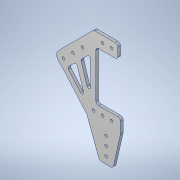
# Autodesk Inventor part: オムニ_後ろ側板
Saved by Autodesk Inventor 2021 (Build 250183000, 183)
## iProperties
Created: 2021-12-02
Part Number: オムニ_後ろ側板
Material: アルミニウム 6061
Document SubType Name: Modeling
Designer: 堀川皓史
Density: 2.7 g/cm^3
Appearance: アルミニウム - フラット
Author: 堀川皓史
Autodesk Inventor part; units mm, degrees
ref_plane "YZ Plane" through (0, 0, 0) normal (1, 0, 0) x (0, 1, 0)
ref_plane "XZ Plane" through (0, 0, 0) normal (0, 1, 0) x (-1, 0, 0)
ref_plane "XY Plane" through (0, 0, 0) normal (0, 0, 1) x (1, 0, 0)
sketch "スケッチ1" plane through (0, 0, 0) normal (0, 0, 1) x (1, 0, 0)
  line L0 (67.5, 17.5) -> (-67.5, 17.5) construction
  line L1 (-67.5, 17.5) -> (-67.5, -17.5) construction
  line L2 (-67.5, -17.5) -> (67.5, -17.5) construction
  line L3 (67.5, -17.5) -> (67.5, 17.5) construction
  line L4 (67.5, 17.5) -> (-67.5, -17.5) construction
  line L5 (-67.5, 17.5) -> (67.5, -17.5) construction
  circle A0 centre (-60, 35) radius 1.6
  circle A1 centre (-70, 35) radius 1.6
  line L6 (-77.5, 27.5) -> (-53, 27.5)
  line L7 (-53, 27.5) -> (-53, 42.5)
  line L8 (-53, 42.5) -> (-80, 42.5) construction
  line L9 (-77.5, 27.5) -> (-77.5, -27.5)
  line L10 (-77.5, -27.5) -> (-50, -27.5)
  circle A2 centre (-60, -35) radius 1.6
  circle A3 centre (-70, -35) radius 1.6
  circle A4 centre (-80, -35) radius 1.6
  line L11 (124.2308, -31.7536) -> (484.5935, -392.1164)
  line L12 (484.5935, -392.1164) -> (488.7129, -553.575)
  line L13 (-80, 21.2868) -> (-468.838, -367.5512) construction
  line L14 (-468.838, -367.5512) -> (-479.4446, -356.9446)
  line L15 (-479.4446, -356.9446) -> (-90.6066, 31.8934) construction
  line L16 (-90.6066, 31.8934) -> (-80, 21.2868) construction
  line L17 (-80, 42.5) -> (-80, 5.3052) construction
  circle A5 centre (-92.3744, 19.519) radius 1.6
  circle A6 centre (-102.981, 8.9124) radius 1.6
  circle A7 centre (-113.5876, -1.6942) radius 1.6
  line L18 (-92.3744, 19.519) -> (-113.5876, -1.6942) construction
  circle A8 centre (-433.75, -321.8566) radius 1.6
  circle A9 centre (-421.9492, -310.0558) radius 1.6
  line L19 (-388.4374, -772.2067) -> (-358.1265, -754.7067) construction
  line L20 (-358.1265, -754.7067) -> (-425.6265, -637.7933) construction
  line L21 (-455.9374, -655.2933) -> (-358.1265, -754.7067) construction
  line L22 (-388.4374, -772.2067) -> (-425.6265, -637.7933) construction
  line L23 (-455.9374, -655.2933) -> (-388.4374, -772.2067) construction
  line L24 (-425.6265, -637.7933) -> (-455.9374, -655.2933) construction
  line L25 (455.9374, -655.2933) -> (425.6265, -637.7933) construction
  line L26 (425.6265, -637.7933) -> (358.1265, -754.7067) construction
  line L27 (388.4374, -772.2067) -> (425.6265, -637.7933) construction
  line L28 (455.9374, -655.2933) -> (358.1265, -754.7067) construction
  line L29 (388.4374, -772.2067) -> (455.9374, -655.2933) construction
  line L30 (358.1265, -754.7067) -> (388.4374, -772.2067) construction
  line L31 (0, 0) -> (0, -263.4473) construction
  line L32 (67.5, 17.5) -> (67.5, -17.5) construction
  circle A10 centre (60, 35) radius 1.6
  circle A11 centre (70, 35) radius 1.6
  line L33 (77.5, 27.5) -> (53, 27.5)
  line L34 (53, 27.5) -> (53, 42.5)
  line L35 (53, 42.5) -> (80, 42.5)
  line L36 (77.5, 27.5) -> (77.5, -27.5)
  line L37 (77.5, -27.5) -> (50, -27.5)
  line L38 (50, -27.5) -> (72.3664, -42.5)
  line L39 (72.3664, -42.5) -> (99.3664, -42.5)
  circle A12 centre (60, -35) radius 1.6
  circle A13 centre (70, -35) radius 1.6
  circle A14 centre (80, -35) radius 1.6
  line L40 (80, 42.5) -> (80, 5.3052) construction
  line L41 (-483.838, -367.5512) -> (-468.838, -367.5512)
  line L42 (-468.838, -367.5512) -> (-468.838, -648.3077)
  line L43 (-468.838, -648.3077) -> (-483.838, -648.3077)
  line L44 (-483.838, -648.3077) -> (-483.838, -367.5512)
  line L45 (-283.2277, -604.4352) -> (-262.2277, -640.8083) construction
  line L46 (345.2492, -497.0108) -> (305.7786, -565.3759) construction
  line L47 (265.1134, -631.6538) -> (-234.8866, -631.6538) construction
  line L48 (-234.8866, -631.6538) -> (-234.8866, -1131.6538) construction
  line L49 (-234.8866, -1131.6538) -> (265.1134, -1131.6538) construction
  line L50 (265.1134, -1131.6538) -> (265.1134, -631.6538) construction
  line L51 (265.1134, -631.6538) -> (-234.8866, -1131.6538) construction
  line L52 (-234.8866, -631.6538) -> (265.1134, -1131.6538) construction
  line L53 (-12.841, -157.5) -> (15.1134, -157.5) construction
  circle A15 centre (1.1362, -409.4569) radius 212.5 construction
  line L54 (501.1362, 53.616) -> (-498.8638, 53.616) construction
  line L55 (-498.8638, 53.616) -> (-498.8638, -946.384) construction
  line L56 (-498.8638, -946.384) -> (501.1362, -946.384) construction
  line L57 (501.1362, -946.384) -> (501.1362, 53.616) construction
  line L58 (501.1362, 53.616) -> (-498.8638, -946.384) construction
  line L59 (-498.8638, 53.616) -> (501.1362, -946.384) construction
  circle A16 centre (1.1362, -409.4569) radius 250 construction
  line L60 (-80, 42.5) -> (-90.6066, 31.8934) construction
  line L61 (-80, 42.5) -> (-118.8909, 3.6091)
  line L62 (-118.8909, -6.9975) -> (-113.5876, -12.3008)
  line L63 (-113.5876, -12.3008) -> (-87.5, -42.5)
  arc A17 (-118.8909, 3.6091) -> (-118.8909, -6.9975) centre (-113.5876, -1.6942) ccw
  line L64 (-80, 42.5) -> (-53, 42.5)
  circle A18 centre (-66, -52.5) radius 1.6
  circle A19 centre (-66, -62.5) radius 1.6
  circle A20 centre (-66, -72.5) radius 1.6
  line L65 (-58.5, -80) -> (-73.5, -80)
  line L66 (-73.5, -80) -> (-87.5, -42.5)
  line L67 (-50, -27.5) -> (-50, -42.5)
  line L68 (-50, -42.5) -> (-58.5, -80)
  point P0 (0, -470)
  point P1 (-102.981, 8.9124)
  point P2 (-77.5, 0)
  point P3 (-407.0319, -705)
  point P4 (-407.0319, -705)
  point P5 (407.0319, -705)
  point P6 (407.0319, -705)
  point P7 (77.5, 0)
  point P8 (15.1134, -881.6538)
  point P9 (1.1362, -446.384)
  point P10 (-124.1942, -1.6942)
  dimension "d27" = 135
  dimension "d28" = 35
  dimension "d29" = 3.2
  dimension "d30" = 3.2
  dimension "d31" = 10
  dimension "d32" = 15
  dimension "d33" = 10
  dimension "d34" = 7.5
  dimension "d35" = 7
  dimension "d36" = 70
  dimension "d37" = 3.2
  dimension "d38" = 3.2
  dimension "d39" = 3.2
  dimension "d40" = 10
  dimension "d41" = 10
  dimension "d45" = 10
  dimension "d46" = 10
  dimension "d53" = 135
  dimension "d54" = 15
  dimension "d55" = 10
  dimension "d57" = 3.2
  dimension "d58" = 3.2
  dimension "d59" = 3.2
  dimension "d60" = 10
  dimension "d61" = 15
  dimension "d62" = 15
  dimension "d63" = 7.5
  dimension "d64" = 45
  dimension "d65" = 3.2
  dimension "d66" = 3.2
  dimension "d69" = 360
  dimension "d76" = 470
  dimension "d77" = 15
  dimension "d80" = 500
  dimension "d81" = 500
  dimension "d82" = 200
  dimension "d83" = 425
  dimension "d84" = 1000
  dimension "d85" = 1000
  dimension "d88" = 42
  dimension "d89" = 500
  dimension "d90" = 7.5
  dimension "d91" = 7.5
  dimension "d112" = 3.2
  dimension "d113" = 3.2
  dimension "d114" = 3.2
  dimension "d115" = 10
  dimension "d116" = 10
  dimension "d117" = 25
  dimension "d118" = 66
  dimension "d120" = 7.5
  dimension "d121" = 7.5
  dimension "d122" = 7.5
  dimension "d123" = 7.5
  dimension "d124" = 7.5
  dimension "d129" = 10
  dimension "d130" = 7.5
  dimension "d131" = 7.5
  constraints: 138 end point, 21 centre point, 14 midpoint, 14 symmetric about line, 11 parallel, 9 perpendicular, 8 horizontal, 5 point on line, 4 vertical, 4 vertical alignment, 3 coincident, 3 horizontal alignment, 2 point on circle, 2 tangent, 1 collinear, 42 other
  measures "d27" distance of L2.end L1.end
  measures "d28" distance of L1.end L0.end
  measures "d29" diameter of A0
  measures "d30" diameter of A1
  measures "d31" distance of A0.centre A1.centre
  measures "d32" distance between parallel lines of L6 L8
  measures "d33" distance between parallel lines of L0 L6
  measures "d34" distance from line of L6 A0.centre
  measures "d35" distance from line of L7 A0.centre
  measures "d36" horizontal distance of A1.centre point (0, 0)
  measures "d37" diameter of A2
  measures "d38" diameter of A3
  measures "d39" diameter of A4
  measures "d40" distance of A3.centre A4.centre
  measures "d41" distance of A2.centre A3.centre
  measures "d45" distance between parallel lines of L10 L2
  measures "d46" distance between parallel lines of L9 L1
  measures "d53" angle of L2 L11
  measures "d54" distance of L13.end L14.end
  measures "d55" distance from line of A1.centre L17
  measures "d57" diameter of A5
  measures "d58" diameter of A6
  measures "d59" diameter of A7
  measures "d60" distance from line of L16 L18.start
  measures "d61" distance of A6.centre L18.start
  measures "d62" distance of L18.end A6.centre
  measures "d63" distance between parallel lines of L13 L18
  measures "d64" angle of L9 L13
  measures "d65" diameter of A8
  measures "d66" diameter of A9
  measures "d76" distance of point (0, -470) point (-407.032, -705)
  measures "d77" distance of L42.end L43.end
  measures "d80" distance of L49.end L48.end
  measures "d81" distance of L48.end L47.end
  measures "d82" distance from line of L53.end L8
  measures "d83" diameter of A15
  measures "d84" distance of L56.end L55.end
  measures "d85" distance of L55.end L54.end
  measures "d88" distance of L45.start L45.end
  measures "d89" diameter of A16
  measures "d90" distance from line of L62 L18.end
  measures "d91" radius of A17
  measures "d112" diameter of A18
  measures "d113" diameter of A19
  measures "d114" diameter of A20
  measures "d115" distance of A19.centre A18.centre
  measures "d116" distance of A20.centre A19.centre
  measures "d117" distance from line of L10 A18.centre
  measures "d118" distance from line of L31 A18.centre
  measures "d120" distance from line of A20.centre L65
  measures "d121" horizontal distance of L63.end A4.centre
  measures "d122" horizontal distance of A4.centre L63.end
  measures "d123" distance from line of L10 A4.centre
  measures "d124" horizontal distance of A20.centre L65.end
  measures "d129" distance from line of A2.centre L67
  measures "d130" horizontal distance of A20.centre L65.start
  measures "d131" vertical distance of A2.centre L67.end
extrude "押し出し1" add sketch "スケッチ1" along normal blind 3 contours L9 L10 L67 L68 L65 L66 L63 L62 A17 L61 L64 L7 L6
fillet "フィレット1" radius 3 10 edges at (-113.5876, -12.3008, 1.5) (-50, -27.5, 1.5) (-77.5, -27.5, 1.5) (-77.5, 27.5, 1.5) (-53, 27.5, 1.5) (-53, 42.5, 1.5) (-80, 42.5, 1.5) (-87.5, -42.5, 1.5) (-73.5, -80, 1.5) (-58.5, -80, 1.5)
sketch "スケッチ2" plane through (0, 0, 3) normal (0, 0, 1) x (1, 0, 0)
  line L0 (-108.1182, -9.4538) -> (-94.6826, -25.0069)
  line L1 (-83.5, -14.6862) -> (-83.5, 12.9584)
  line L2 (-86.9142, 14.3726) -> (-93.4726, 7.8142)
  line L3 (-77.5, -24.5) -> (-77.5, 24.5) projected
  line L4 (-80.8787, 41.6213) -> (-118.8909, 3.6091) projected
  line L5 (-113.516, -12.3836) -> (-87.852, -42.0925) projected
  line L6 (-96.7234, 4.5634) -> (-83.5, -37.9521) construction
  line L7 (-98.1366, -0.994) -> (-91.2594, -23.1055)
  line L8 (-93.9681, 5.806) -> (-87.4098, -15.2802)
  line L9 (-101.4606, -0.1738) -> (-108.019, -6.7322)
  arc A0 (-98.1366, -0.994) -> (-101.4606, -0.1738) centre (-100.0464, -1.588) ccw
  arc A1 (-93.4726, 7.8142) -> (-93.9681, 5.806) centre (-92.0583, 6.4) ccw
  arc A2 (-94.6826, -25.0069) -> (-91.2594, -23.1055) centre (-93.1692, -23.6995) ccw
  arc A3 (-87.4098, -15.2802) -> (-83.5, -14.6862) centre (-85.5, -14.6862) ccw
  arc A4 (-83.5, 12.9584) -> (-86.9142, 14.3726) centre (-85.5, 12.9584) ccw
  arc A5 (-108.019, -6.7322) -> (-108.1182, -9.4538) centre (-106.6047, -8.1464) ccw
  line L10 (-53, -27.5) -> (-74.5, -27.5) projected
  point P0 (0, 0)
  point P1 (-99.1198, 2.167)
  dimension "d95" = 6
  dimension "d97" = 15
  dimension "d98" = 6
  dimension "d99" = 3
  dimension "d100" = 3
  dimension "d101" = 2
  dimension "d102" = 2
  constraints: 14 end point, 12 point on circle, 12 tangent, 7 point on line, 6 centre point, 5 parallel, 4 equal radius, 1 collinear, 1 vertical
  measures "d95" distance between parallel lines of L3 L1
  measures "d97" distance between parallel lines of L4 L2
  measures "d98" distance between parallel lines of L5 L0
  measures "d99" distance between parallel lines of L6 L8
  measures "d100" distance between parallel lines of L6 L7
  measures "d101" radius of A0
  measures "d102" radius of A2
extrude "押し出し2" cut sketch "スケッチ2" against normal blind 3
